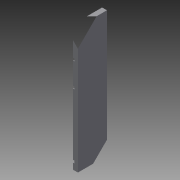
# Autodesk Inventor part: Yagi_BaseFrame
Saved by Autodesk Inventor 2014 (Build 180170000, 170)
## iProperties
Created: 2015-01-07
Part Number: Yagi_BaseFrame
Material: Generic
Document SubType Name: Modeling
Designer: Owner
Density: 1 g/cm^3
Appearance: Default
Author: Owner
Autodesk Inventor part; units mm, degrees
ref_plane "YZ Plane" through (0, 0, 0) normal (1, 0, 0) x (0, 1, 0)
ref_plane "XZ Plane" through (0, 0, 0) normal (0, 1, 0) x (-1, 0, 0)
ref_plane "XY Plane" through (0, 0, 0) normal (0, 0, 1) x (1, 0, 0)
sketch "Sketch1" plane through (0, 0, 0) normal (0, 0, 1) x (1, 0, 0)
  line L0 (62.0733, 80.7499) -> (62.0733, -84.3501)
  line L1 (68.4233, 80.7499) -> (68.4233, -84.3501)
  line L2 (62.0733, 42.6499) -> (63.6608, 42.6499)
  line L3 (63.6608, 42.6499) -> (63.6608, 39.4749)
  line L4 (63.6608, 39.4749) -> (62.0733, 39.4749)
  line L5 (62.0733, 39.4749) -> (62.0733, 42.6499)
  line L6 (62.0733, -84.3501) -> (68.4233, -84.3501)
  line L7 (62.0733, 80.7499) -> (68.4233, 80.7499)
  line L8 (62.0733, 10.8999) -> (63.6608, 10.8999)
  line L9 (63.6608, 10.8999) -> (63.6608, 7.7249)
  line L10 (63.6608, 7.7249) -> (62.0733, 7.7249)
  line L11 (62.0733, 7.7249) -> (62.0733, 10.8999)
  line L12 (62.0733, -76.2221) -> (63.6608, -76.2221)
  line L13 (63.6608, -76.2221) -> (63.6608, -73.0471)
  line L14 (63.6608, -73.0471) -> (62.0733, -73.0471)
  line L15 (62.0733, -73.0471) -> (62.0733, -76.2221)
  point P0 (0, 0)
  dimension "d1" = 165.1
  dimension "d2" = 6.35
  dimension "d8" = 3.175
  dimension "d9" = 1.5875
  dimension "d14" = 3.175
  dimension "d15" = 1.5875
  dimension "d16" = 3.175
  dimension "d17" = 1.5875
  dimension "d18" = 87.122
  dimension "d19" = 28.575
  dimension "d20" = 38.1
  constraints: 32 end point, 7 parallel, 4 perpendicular, 3 horizontal, 3 point on line
  measures "d1" distance of L0.start L0.end
  measures "d2" distance between parallel lines of L1 L0
  measures "d8" distance of L2.end L3.end
  measures "d9" distance of L2.start L2.end
  measures "d14" distance of L8.end L9.end
  measures "d15" distance of L8.start L8.end
  measures "d16" distance of L12.end L13.end
  measures "d17" distance of L13.end L14.end
  measures "d18" distance between parallel lines of L12 L8
  measures "d19" distance between parallel lines of L4 L8
  measures "d20" distance between parallel lines of L7 L2
extrude "Extrusion1" add sketch "Sketch1" along normal blind 38.1 contours L7 L1 L6 L0 L12 L13 L14 L10 L9 L8 L4 L3 L2
body "Solid1"
